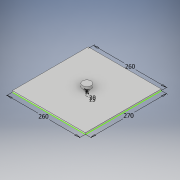
# Autodesk Inventor part: Part Buttom
Saved by Autodesk Inventor 2019 (Build 230136000, 136)
## iProperties
Created: 2019-07-08
Part Number: Part Buttom
Material: Generic
Document SubType Name: Modeling
Designer: azriel
Density: 1 g/cm^3
Appearance: Default
Author: azriel
Autodesk Inventor part; units mm, degrees
ref_plane "YZ Plane" through (0, 0, 0) normal (1, 0, 0) x (0, 1, 0)
ref_plane "XZ Plane" through (0, 0, 0) normal (0, 1, 0) x (-1, 0, 0)
ref_plane "XY Plane" through (0, 0, 0) normal (0, 0, 1) x (1, 0, 0)
sketch "Sketch1" plane through (0, 0, 0) normal (0, 1, 0) x (-1, 0, 0)
  line L0 (-138.1445, 75.4197) -> (-138.1445, 125.4197)
  line L1 (-138.1445, -54.5803) -> (-138.1445, -4.5803)
  line L2 (-118.1445, -74.5803) -> (-68.1445, -74.5803)
  line L3 (1.8555, -74.5803) -> (51.8555, -74.5803)
  line L4 (71.8555, -54.5803) -> (71.8555, -4.5803)
  line L5 (71.8555, 125.4197) -> (71.8555, 75.4197)
  line L6 (51.8555, 145.4197) -> (1.8555, 145.4197)
  line L7 (-68.1445, 145.4197) -> (-118.1445, 145.4197)
  line L8 (51.8555, -74.5803) -> (71.8555, -74.5803)
  line L9 (71.8555, -74.5803) -> (71.8555, -54.5803)
  line L10 (71.8555, -74.5803) -> (-138.1445, -74.5803)
  line L11 (-138.1445, -74.5803) -> (-138.1445, 145.4197)
  line L12 (-138.1445, 145.4197) -> (71.8555, 145.4197)
  line L13 (71.8555, 145.4197) -> (71.8555, -74.5803)
  line L14 (96.8555, -89.5803) -> (96.8555, -99.5803)
  line L15 (96.8555, -99.5803) -> (-163.1445, -99.5803)
  line L16 (-163.1445, -99.5803) -> (-163.1445, 170.4197)
  line L17 (-163.1445, 170.4197) -> (96.8555, 170.4197)
  line L18 (96.8555, 170.4197) -> (96.8555, -99.5803)
  circle A0 centre (-33.1445, 35.4197) radius 7.5
  circle A1 centre (-33.1445, 35.4197) radius 15
  point P0 (0, 0)
  dimension "d37" = 260
  dimension "d38" = 270
  dimension "d39" = 260
  dimension "d40" = 15
  dimension "d41" = 30
  constraints: 38 end point, 6 horizontal, 3 perpendicular, 2 centre point, 2 point on line, 2 vertical, 1 coincident, 1 collinear
  measures "d37" distance of L14.end L15.end
  measures "d38" distance of L15.end L16.end
  measures "d39" distance of L16.end L17.end
  measures "d40" diameter of A0
  measures "d41" diameter of A1
extrude "Extrusion2" add sketch "Sketch1" against normal blind 5 contours L0 L11 L12 L7 L6 L13 L5 L4 L9 L8 L3 L10 L2 L1 | A0 | A1
extrude "Extrusion3" add sketch "Sketch1" along normal blind 5 contours L0 L11 L12 L7 L6 L13 L5 L4 L9 L8 L3 L10 L2 L1 | L14 L15 L16 L17 L18 | A0 | A1
extrude "Extrusion4" add sketch "Sketch1" along normal blind 15 contours A0
ref_plane "Work Plane3" through (33.1445, 15, 35.4197) normal (0, 1, 0) x (1, 0, 0)
sketch "Sketch2" plane through (33.1445, 15, 35.4197) normal (0, 1, 0) x (1, 0, 0)
  circle A0 centre (0, 0) radius 15
  point P0 (-33.1445, 35.4197)
  dimension "d53" = 30
  constraints: 1 centre point
  measures "d53" diameter of A0
extrude "Extrusion6" add sketch "Sketch2" along normal blind 10
body "Solid2"
